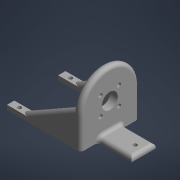
# Autodesk Inventor part: V2 5202 Series Yellow Jacket planetary Gear Motor Mount
Saved by Autodesk Inventor 2022 (Build 260153000, 153)
## iProperties
Part Number: V2 5202 Series Yellow Jacket planetary Gear Motor Mount
Material: Generic
Document SubType Name: Modeling
Designer: izack
Appearance: Default
Author: izack
## iProperties of the stored document V2 5202 Series Yellow Jacket planetary Gear Motor Mount_3DPrint.ipt
Part Number: V2 5202 Series Yellow Jacket planetary Gear Motor Mount_3DPrint
Material: Generic
Document SubType Name: Modeling
Designer: izack
Appearance: Default
Author: izack
Autodesk Inventor part; units mm, degrees
ref_plane "YZ Plane" through (0, 0, 0) normal (1, 0, 0) x (0, 1, 0)
ref_plane "XZ Plane" through (0, 0, 0) normal (0, 1, 0) x (-1, 0, 0)
ref_plane "XY Plane" through (0, 0, 0) normal (0, 0, 1) x (1, 0, 0)
sketch "Sketch1" plane through (0, 0, 0) normal (0, 1, 0) x (-1, 0, 0)
  line L0 (0, 0) -> (93.5, 0)
  line L1 (93.5, 0) -> (93.5, -50.8)
  line L2 (93.5, -50.8) -> (0, -50.8)
  line L3 (0, -50.8) -> (0, 0)
  line L4 (0, -15) -> (29.5, -15)
  line L5 (0, -35.8) -> (29.5, -35.8)
  circle A0 centre (7.5, -25.4) radius 1.7
  line L6 (29.5, 0) -> (29.5, -50.8)
  line L7 (35.85, 0) -> (35.85, -50.8)
  line L8 (93.5, -6.35) -> (35.85, -6.35)
  line L9 (93.5, -44.45) -> (35.85, -44.45)
  circle A1 centre (86, -3.175) radius 1.7
  circle A2 centre (86, -47.62) radius 1.7
  line L10 (93.5, -3.175) -> (67.2869, -3.175) construction
  line L11 (93.5, -25.4) -> (0, -25.4) construction
  line L12 (93.5, -47.62) -> (77.4227, -47.62) construction
  dimension "d0" = 93.5
  dimension "d1" = 50.8
  dimension "d2" = 15
  dimension "d3" = 15
  dimension "d4" = 3.4
  dimension "d5" = 7.5
  dimension "d6" = 22
  dimension "d7" = 6.35
  dimension "d8" = 6.35
  dimension "d9" = 6.35
  dimension "d10" = 3.4
  dimension "d11" = 3.4
  dimension "d12" = 3.18
  dimension "d13" = 3.175
  dimension "d14" = 7.5
  dimension "d15" = 7.5
  constraints: 26 end point, 16 point on line, 5 perpendicular, 4 horizontal, 3 centre point, 3 parallel, 2 midpoint
  measures "d0" distance of L1.end L2.end
  measures "d1" distance of L0.end L1.end
  measures "d2" distance between parallel lines of L2 L5
  measures "d3" distance between parallel lines of L0 L4
  measures "d4" diameter of A0
  measures "d5" distance from line of L3 A0.centre
  measures "d6" distance from line of L6 A0.centre
  measures "d7" distance between parallel lines of L6 L7
  measures "d8" distance between parallel lines of L2 L9
  measures "d9" distance between parallel lines of L0 L8
  measures "d10" diameter of A1
  measures "d11" diameter of A2
  measures "d12" distance between parallel lines of L2 L12
  measures "d13" distance between parallel lines of L0 L10
  measures "d14" distance from line of L1 A2.centre
  measures "d15" distance from line of L1 A1.centre
extrude "Extrusion1" add sketch "Sketch1" along normal blind 4 contours L0 L7 L2 L6 | L4 L6 L5 L3 | L0 L1 L8 L7 | L9 L1 L2 L7
sketch "Sketch2" plane through (-29.5, 0, -35.8) normal (1, 0, 0) x (0, 0, -1)
  line L0 (-20.8, 4) -> (0, 4) projected
  line L1 (-10.4, 4) -> (-10.4, 39.8129) construction
  circle A0 centre (-10.4, 26.1951) radius 6.86
  line L2 (-29.45, 4) -> (-35.8, 4) projected
  line L3 (0, 4) -> (15, 4) projected
  line L4 (-35.8, 4) -> (15, 4)
  circle A1 centre (-18.4, 34.1377) radius 1.7
  line L5 (-18.4, 18.2526) -> (-2.4, 18.2526) construction
  line L6 (-2.4, 18.2526) -> (-2.4, 34.1377) construction
  line L7 (-2.4, 34.1377) -> (-18.4, 34.1377) construction
  line L8 (-18.4, 34.1377) -> (-18.4, 18.2526) construction
  line L9 (-18.4, 18.2526) -> (-2.4, 34.1377) construction
  line L10 (-2.4, 18.2526) -> (-18.4, 34.1377) construction
  circle A2 centre (-2.4, 34.1377) radius 1.7
  line L11 (-18.4, 26.1951) -> (-2.4, 26.1951) construction
  circle A3 centre (-18.4, 18.2526) radius 1.7
  circle A4 centre (-2.4, 18.2526) radius 1.7
  line L12 (-35.8, 4) -> (-35.8, 51.4128)
  line L13 (15, 4) -> (15, 51.4128)
  circle A5 centre (-10.4, 26.1951) radius 25.4
  point P0 (-35.8, 0)
  point P1 (-29.45, 4)
  point P2 (15, 26.1951)
  point P3 (-35.8, 26.1951)
  dimension "d18" = 13.72
  dimension "d20" = 3.4
  dimension "d22" = 16
  constraints: 22 end point, 6 centre point, 4 coincident, 3 midpoint, 3 symmetric about line, 3 vertical, 2 parallel, 1 collinear, 1 horizontal, 1 perpendicular, 1 point on line, 3 other
  measures "d18" diameter of A0
  measures "d20" diameter of A1
  measures "d22" distance of L7.end L6.end
extrude "Extrusion2" add sketch "Sketch2" against normal up to surface (6.35 mm away) contours L4 A5 L3 L0 | L4 L2 L12 A5 | A5 L13 L3 picked at (-8.0552, 8.2845)
chamfer "Chamfer1" distance 44.5 distance2 25.25 1 edges at (-35.85, 4, -3.175) measured on face at (-36.35, 4, -3.175)
chamfer "Chamfer2" distance 44.5 distance2 25.25 1 edges at (-35.85, 4, -47.625) measured on face at (-36.35, 4, -47.625)
fillet "Fillet1" radius 3 16 edges at (-29.5, 13.0976, 0) (-29.5, 13.0976, -50.8) (-29.5, 51.5951, -25.4) (-35.85, 51.5951, -25.4) (-29.5, 2, -35.8) (-29.5, 4, -25.4) (-29.5, 2, -15) (-14.75, 4, -15) (0, 4, -25.4) (-14.75, 4, -35.8) (-38.537, 27.7254, -50.7539) (-60.7919, 15.0976, -50.8) (-58.1, 16.625, -44.45) (-58.1, 16.625, -6.35) (-38.537, 27.7254, -0.0461) (-60.7919, 15.0976, 0)
body "Solid1"
